Autodesk Fusion 360 part; units mm, degrees
note: some values were not read from the file. Set by a fixed rule: which sketch regions a step uses.
(part 2 of 2)
extrude "Extrude7" add sketch "Sketch3" against normal blind 4 contours A0 | A2 | A4 | A6 bodies 11 in component "bottom"
sketch "Sketch4" plane through (0, 0, 17.5) normal (0, 0, -1) x (1, 0, 0) in component "bottom"
  line L0 (73, -115.5) -> (73, -139.5)
  line L1 (73, -139.5) -> (27, -139.5)
  line L2 (27, -139.5) -> (27, -115.5)
  line L3 (27, -115.5) -> (73, -115.5)
  line L4 (25, -141.5) -> (75, -141.5)
  line L5 (75, -141.5) -> (75, -113.5)
  line L6 (75, -113.5) -> (25, -113.5)
  line L7 (25, -113.5) -> (25, -141.5)
  circle A0 centre (30.95, -119.25) radius 2.5
  circle A1 centre (30.95, -119.25) radius 1.4
  circle A2 centre (69.05, -119.25) radius 2.5
  circle A3 centre (69.05, -119.25) radius 1.4
  circle A4 centre (69.05, -135.75) radius 2.5
  circle A5 centre (69.05, -135.75) radius 1.4
  circle A6 centre (30.95, -135.75) radius 2.5
  circle A7 centre (30.95, -135.75) radius 1.4
extrude "Extrude8" add sketch "Sketch4" against normal blind 7 contours L0 L1 L2 L3 bodies 12 in component "bottom"
extrude "Extrude9" add sketch "Sketch4" against normal blind 4 contours A0 | A2 | A4 | A6 bodies 12 in component "bottom"
extrude "Extrude10" add sketch "Sketch1 (2)" against normal blind 4 contours A99 A102 L91 A128 A132 L174 | A99 L88 A100 A128 A134 L175 | A127 A128 L174 A137 L175 | A128 A132 A133 A134 L173 L174 L175 L176 | A127 A128 L174 A137 L175 | A101 L90 A102 A132 A133 L173 | A131 A132 L173 A136 L174 | A131 A132 L173 A136 L174 | A129 A134 L175 A138 L176 | A129 A134 L175 A138 L176 | A100 L89 A101 A133 A134 L176 | A127 A137 | A127 A137 | A130 A133 A135 L173 L176 | A130 A133 A135 L173 L176 | A131 A136 | A131 A136 | A129 A138 | A129 A138 | A130 A135 | A130 A135 | L93 L96 L136 L137 | L93 L96 L99 L100 L104 L115 | L93 L115 L136 L137 | L96 L104 L136 L137 | L93 L113 L115 L116 L117 | L93 L100 L113 L114 L115 L117 | L103 L109 L112 L116 L119 L123 L128 L132 L134 L135 L136 L137 L138 L139 L140 L141 | L96 L99 L102 L104 L105 | L96 L102 L103 L104 L106 | L93 L111 L112 L113 L117 | L93 L100 L110 L111 L113 L117 | L96 L99 L102 L107 L172 | L96 L102 L106 L107 L108 L109 | L93 L111 L138 L139 | L93 L94 L100 L101 L111 L120 | L95 L96 L98 L99 L127 L172 | L96 L108 L134 L135 | L93 L94 L138 L139 | L95 L96 L134 L135 | L94 L120 L138 L139 | L95 L127 L134 L135 | L94 L118 L119 L120 L122 | L94 L101 L118 L120 L121 L122 | L95 L127 L128 L129 L133 | L95 L98 L126 L127 L129 L133 | L94 L118 L122 L123 L124 | L94 L101 L118 L122 L124 L125 | L95 L129 L131 L132 L133 | L95 L98 L129 L130 L131 L133 | L94 L95 L124 L140 | L94 L95 L98 L101 L124 L131 | L95 L131 L140 L141 | L154 L155 L156 L157 | L159 L160 L162 L163 bodies 2 3 4 5 6 7 8 9 10 11 12 in component "bottom"
sketch "Sketch5" plane through (175, 0, 0) normal (1, 0, 0) x (0, 1, 0) in component "bottom"
  line L0 (6, 56.5) -> (6, -2.5)
  line L1 (6, -2.5) -> (139, -2.5)
  line L2 (139, -2.5) -> (139, 56.5)
  line L3 (126, -17.5) -> (96, -17.5) construction
  line L4 (96, -17.5) -> (111, -17.5) construction
  line L5 (111, -17.5) -> (111, 50.5) construction
  line L6 (139, 56.5) -> (6, 56.5)
  line L7 (141.5, 52.5) -> (113.5, 52.5)
  line L8 (113.5, 52.5) -> (141.5, 52.5)
  line L9 (0, 52.5) -> (6.7574, 52.5)
  line L10 (6.4384, 52.5) -> (138.5616, 52.5)
  line L11 (138.2426, 52.5) -> (145, 52.5)
  line L12 (138.2426, 52.5) -> (145, 52.5)
  line L13 (138.5616, 52.5) -> (6.4384, 52.5)
  line L14 (0, 52.5) -> (6.7574, 52.5)
  line L15 (30.523, 52.5) -> (6.123, 52.5)
  line L16 (6.123, 52.5) -> (13.123, 52.5)
  line L17 (13.123, 52.5) -> (30.523, 52.5)
  line L18 (30.523, 52.5) -> (13.123, 52.5)
  line L19 (13.123, 52.5) -> (6.123, 52.5)
  line L20 (6.123, 52.5) -> (30.523, 52.5)
  line L21 (70.523, 52.5) -> (63.523, 52.5)
  line L22 (63.523, 52.5) -> (46.123, 52.5)
  line L23 (46.123, 52.5) -> (70.523, 52.5)
  line L24 (46.123, 52.5) -> (63.523, 52.5)
  line L25 (63.523, 52.5) -> (70.523, 52.5)
  line L26 (70.523, 52.5) -> (46.123, 52.5)
  line L27 (80.5, 52.5) -> (108.5, 52.5)
  line L28 (108.5, 52.5) -> (80.5, 52.5)
  line L29 (111, 50.5) -> (111, 52.5)
  line L30 (111, 52.5) -> (111, 25.5)
  circle A0 centre (126, 25.5) radius 3.2
  line L31 (105, 22) -> (97, 22)
  line L32 (95, 24) -> (95, 27)
  line L33 (97, 29) -> (105, 29)
  line L34 (107, 27) -> (107, 24)
  line L35 (107, 22) -> (95, 29) construction
  line L36 (101, 25.5) -> (91, 25.5) construction
  line L37 (101, 25.5) -> (111, 25.5) construction
  circle A1 centre (91, 25.5) radius 1.65
  circle A2 centre (111, 25.5) radius 1.65
  arc A3 (105, 22) -> (107, 24) centre (105, 24) ccw
  arc A4 (107, 27) -> (105, 29) centre (105, 27) ccw
  arc A5 (95, 24) -> (97, 22) centre (97, 24) ccw
  arc A6 (97, 29) -> (95, 27) centre (97, 27) ccw
  line L38 (111, 25.5) -> (126, 25.5) construction
  point P0 (126, -17.5)
  point P1 (96, -17.5)
  point P2 (95, 22)
  point P3 (107, 29)
  dimension "d207" = 27
  dimension "d220" = 6.4
  dimension "d221" = 12
  dimension "d222" = 7
  dimension "d223" = 10
  dimension "d224" = 10
  dimension "d225" = 3.3
  dimension "d226" = 3.3
  dimension "d227" = 2
  dimension "d228" = 15
  constraint coincident P0 L3.start
  constraint coincident P1 L3.end
  constraint midpoint L3 L4.end
  constraint coincident L10 L29.end
  constraint perpendicular L10 L29
  constraint collinear L5 L29
  constraint horizontal L31
  constraint vertical L32
  constraint horizontal L33
  constraint vertical L34
  constraint midpoint L35 L36.start
  constraint perpendicular L32 L36
  constraint perpendicular L34 L37
  constraint coincident L36.end A1.centre
  constraint coincident L30.end L37.end
  constraint coincident L35.start L31
  constraint coincident L35.start L34
  constraint tangent L31 A3
  constraint tangent L34 A3
  constraint coincident P3 L33
  constraint coincident P3 L34
  constraint tangent L33 A4
  constraint tangent L34 A4
  constraint equal A3 A4
  constraint coincident P2 L31
  constraint coincident P2 L32
  constraint tangent L31 A5
  constraint tangent L32 A5
  constraint equal A3 A5
  constraint coincident L35.end L33
  constraint coincident L35.end L32
  constraint tangent L33 A6
  constraint tangent L32 A6
  constraint equal A3 A6
  constraint parallel L37 L38
  constraint coincident A0.centre L38.end
  constraint perpendicular L27 L30
  measures "d207" distance of L29.end L30.end
  measures "d220" diameter of A0
  measures "d221" distance of L35.start P2
  measures "d222" distance of L35.start P3
  measures "d223" distance of L36.start L36.end
  measures "d224" distance of L36.start L30.end
  measures "d225" diameter of A1
  measures "d226" diameter of A2
  measures "d227" radius of A3
  measures "d228" distance of L30.end A0.centre
extrude "Extrude12" add sketch "Sketch4" sketch "Sketch3" along normal blind 4 contours L0 L1 L2 L3 | L4 L5 L6 L7 | A0 | A2 | A4 | A6 of sketch 2 contours L0 L1 L2 L3 | L4 L5 L6 L7 | A0 | A2 | A4 | A6 bodies 2 in component "bottom"
extrude "Extrude13" cut 4 faces at (67.0569, 86.9948, 21.5) (67.0569, 103.4948, 21.5) (29.1251, 85.1561, 21.5) (29.1251, 101.6561, 21.5) along direction (0, 0, -1) blind 4 on bodies 2 bodies 2 in component "bottom"
extrude "Extrude14" cut 1 faces at (44.4008, 96.8884, 24.5) along direction (0, 0, -1) blind 4 on bodies 2 bodies 2 in component "bottom"
extrude "Extrude15" cut 1 faces at (44.4008, 125.1116, 24.5) along direction (0, 0, -1) blind 4 on bodies 2 bodies 2 in component "bottom"
extrude "Extrude16" cut 4 faces at (33.0688, 119.4438, 21.5) (33.0163, 135.2426, 21.5) (67.0569, 119.9948, 21.5) (66.9837, 136.2574, 21.5) along direction (0, 0, -1) blind 4 on bodies 2 bodies 2 in component "bottom"
extrude "Extrude17" cut 1 faces at (141, 75.8333, 56.5) along direction (0, 0, -1) blind 1.5 on bodies 2 bodies 2 in component "bottom"
extrude "Extrude18" cut 1 faces at (58.8128, 145, 34.1667) along direction (0, 1, 0) blind 2.5 on bodies 2 bodies 2 in component "bottom"
extrude "Extrude19" cut 1 faces at (170, 94.5205, 15.8333) along direction (1, 0, 0) blind 2.5 on bodies 2 bodies 2 in component "bottom"
extrude "Extrude20" cut 1 faces at (0, 50.4795, 34.1667) along direction (-1, 0, 0) blind 2.5 on bodies 2 bodies 2 in component "bottom"
extrude "Extrude21" cut 1 faces at (111.1872, 0, 34.1667) along direction (0, -1, 0) blind 2.5 on bodies 2 bodies 2 in component "bottom"
extrude "Extrude22" cut 2 faces at (36.4, 13.123, 35.8333) (63.6, 13.123, 35.8333) along direction (0, -1, 0) blind 2 on bodies 2 bodies 2 in component "bottom"
extrude "Extrude23" cut 2 faces at (63.6, 63.523, 35.8333) (36.4, 63.523, 35.8333) along direction (0, 1, 0) blind 2 on bodies 2 bodies 2 in component "bottom"
extrude "Extrude24" cut 2 faces at (24.8, 52.5896, 35.8333) (24.8, 17.5896, 19.1667) along direction (-1, 0, 0) blind 2 on bodies 2 bodies 2 in component "bottom"
extrude "Extrude25" cut 2 faces at (75.2, 17.5896, 19.1667) (75.2, 52.5896, 35.8333) along direction (1, 0, 0) blind 2 on bodies 2 bodies 2 in component "bottom"
fillet "Fillet3" radius 8 8 edges at (67.5, 65.523, 52.5) (32.5, 65.523, 52.5) (22.8, 55.823, 52.5) (22.8, 20.823, 52.5) (32.5, 11.123, 52.5) (77.2, 20.823, 52.5) (67.5, 11.123, 52.5) (77.2, 55.823, 52.5) on bodies 2 in component "bottom"
fillet "Fillet4" radius 2 8 edges at (50, 113.5, 13.5) (75, 127.5, 13.5) (50, 141.5, 13.5) (25, 127.5, 13.5) (25, 94.5, 13.5) (50, 80.5, 13.5) (50, 108.5, 13.5) (75, 94.5, 13.5) on bodies 2 in component "bottom"
fillet "Fillet5" radius 6 8 edges at (85, 150, 55) (171.7782, 146.7782, 55) (175, 72.5, 55) (171.7782, -1.7782, 55) (85, -5, 55) (-1.7782, -1.7782, 55) (-5, 72.5, 55) (-1.7782, 146.7782, 55) on bodies 2 in component "bottom"
fillet "Fillet6" radius 2 8 edges at (50, 82.5, 55) (27, 94.5, 55) (50, 106.5, 55) (73, 94.5, 55) (50, 115.5, 55) (27, 127.5, 55) (50, 139.5, 55) (73, 127.5, 55) on bodies 2 in component "bottom"
extrude "Extrude6'" add 9 faces at (98.1986, 29.7171, -15.5) (125.1986, 29.7171, -15.5) (98.2222, 58.415, -15.5) (125.2222, 58.415, -15.5) (151.6624, 57.1856, -15.5) (153.6175, 30.3228, -15.5) (125.1986, 2.7171, -15.5) (153.6175, 3.6077, -15.5) (98.1986, 2.7171, -15.5) along direction (0, 0, -1) blind 2 on bodies 1 bodies 1 in component "Lid"
sketch "Sketch2 (2)" plane through (0, 0, -15) normal (0, 0, 1) x (-1, 0, 0) in component "Lid"
  arc A0 (-63, -19.323) -> (-61, -21.323) centre (-61, -19.323) ccw
  line L0 (-63, -19.323) -> (-63, -12.323)
  arc A1 (-61, -10.323) -> (-63, -12.323) centre (-61, -12.323) ccw
  line L1 (-61, -10.323) -> (-54, -10.323)
  arc A2 (-52, -12.323) -> (-54, -10.323) centre (-54, -12.323) ccw
  line L2 (-52, -12.323) -> (-52, -19.323)
  arc A3 (-54, -21.323) -> (-52, -19.323) centre (-54, -19.323) ccw
  line L3 (-54, -21.323) -> (-61, -21.323)
  arc A4 (-78, -19.323) -> (-76, -21.323) centre (-76, -19.323) ccw
  line L4 (-78, -19.323) -> (-78, -12.323)
  arc A5 (-76, -10.323) -> (-78, -12.323) centre (-76, -12.323) ccw
  line L5 (-76, -10.323) -> (-69, -10.323)
  arc A6 (-67, -12.323) -> (-69, -10.323) centre (-69, -12.323) ccw
  line L6 (-67, -12.323) -> (-67, -19.323)
  arc A7 (-69, -21.323) -> (-67, -19.323) centre (-69, -19.323) ccw
  line L7 (-69, -21.323) -> (-76, -21.323)
  arc A8 (-48, -19.323) -> (-46, -21.323) centre (-46, -19.323) ccw
  line L8 (-48, -19.323) -> (-48, -12.323)
  arc A9 (-46, -10.323) -> (-48, -12.323) centre (-46, -12.323) ccw
  line L9 (-46, -10.323) -> (-39, -10.323)
  arc A10 (-37, -12.323) -> (-39, -10.323) centre (-39, -12.323) ccw
  line L10 (-37, -12.323) -> (-37, -19.323)
  arc A11 (-39, -21.323) -> (-37, -19.323) centre (-39, -19.323) ccw
  line L11 (-39, -21.323) -> (-46, -21.323)
  circle A12 centre (-1.7574, -143.2426) radius 1.65
  arc A13 (-78, -64.323) -> (-76, -66.323) centre (-76, -64.323) ccw
  line L12 (-78, -64.323) -> (-78, -57.323)
  arc A14 (-76, -55.323) -> (-78, -57.323) centre (-76, -57.323) ccw
  line L13 (-76, -55.323) -> (-69, -55.323)
  arc A15 (-67, -57.323) -> (-69, -55.323) centre (-69, -57.323) ccw
  line L14 (-67, -57.323) -> (-67, -64.323)
  arc A16 (-69, -66.323) -> (-67, -64.323) centre (-69, -64.323) ccw
  line L15 (-69, -66.323) -> (-76, -66.323)
  arc A17 (-33, -49.323) -> (-31, -51.323) centre (-31, -49.323) ccw
  line L16 (-33, -49.323) -> (-33, -42.323)
  arc A18 (-31, -40.323) -> (-33, -42.323) centre (-31, -42.323) ccw
  line L17 (-31, -40.323) -> (-24, -40.323)
  arc A19 (-22, -42.323) -> (-24, -40.323) centre (-24, -42.323) ccw
  line L18 (-22, -42.323) -> (-22, -49.323)
  arc A20 (-24, -51.323) -> (-22, -49.323) centre (-24, -49.323) ccw
  line L19 (-24, -51.323) -> (-31, -51.323)
  circle A21 centre (-113.5, -77.8144) radius 1.45
  circle A22 centre (-168.2426, -1.7574) radius 1.65
  arc A23 (-48, -49.323) -> (-46, -51.323) centre (-46, -49.323) ccw
  line L20 (-48, -49.323) -> (-48, -42.323)
  arc A24 (-46, -40.323) -> (-48, -42.323) centre (-46, -42.323) ccw
  line L21 (-46, -40.323) -> (-39, -40.323)
  arc A25 (-37, -42.323) -> (-39, -40.323) centre (-39, -42.323) ccw
  line L22 (-37, -42.323) -> (-37, -49.323)
  arc A26 (-39, -51.323) -> (-37, -49.323) centre (-39, -49.323) ccw
  line L23 (-39, -51.323) -> (-46, -51.323)
  circle A27 centre (-125.5, -65.3144) radius 3.75
  line L24 (-138.5, -101.6644) -> (-138.5, -86.6644)
  line L25 (-138.5, -86.6644) -> (-112.5, -86.6644)
  line L26 (-112.5, -86.6644) -> (-112.5, -101.6644)
  line L27 (-112.5, -101.6644) -> (-138.5, -101.6644)
  circle A28 centre (-1.7574, -1.7574) radius 1.65
  arc A29 (-48, -64.323) -> (-46, -66.323) centre (-46, -64.323) ccw
  line L28 (-48, -64.323) -> (-48, -57.323)
  arc A30 (-46, -55.323) -> (-48, -57.323) centre (-46, -57.323) ccw
  line L29 (-46, -55.323) -> (-39, -55.323)
  arc A31 (-37, -57.323) -> (-39, -55.323) centre (-39, -57.323) ccw
  line L30 (-37, -57.323) -> (-37, -64.323)
  arc A32 (-39, -66.323) -> (-37, -64.323) centre (-39, -64.323) ccw
  line L31 (-39, -66.323) -> (-46, -66.323)
  arc A33 (-63, -64.323) -> (-61, -66.323) centre (-61, -64.323) ccw
  line L32 (-63, -64.323) -> (-63, -57.323)
  arc A34 (-61, -55.323) -> (-63, -57.323) centre (-61, -57.323) ccw
  line L33 (-61, -55.323) -> (-54, -55.323)
  arc A35 (-52, -57.323) -> (-54, -55.323) centre (-54, -57.323) ccw
  line L34 (-52, -57.323) -> (-52, -64.323)
  arc A36 (-54, -66.323) -> (-52, -64.323) centre (-54, -64.323) ccw
  line L35 (-54, -66.323) -> (-61, -66.323)
  circle A37 centre (-137.5, -77.8144) radius 1.45
  arc A38 (-63, -34.323) -> (-61, -36.323) centre (-61, -34.323) ccw
  line L36 (-63, -34.323) -> (-63, -27.323)
  arc A39 (-61, -25.323) -> (-63, -27.323) centre (-61, -27.323) ccw
  line L37 (-61, -25.323) -> (-54, -25.323)
  arc A40 (-52, -27.323) -> (-54, -25.323) centre (-54, -27.323) ccw
  line L38 (-52, -27.323) -> (-52, -34.323)
  arc A41 (-54, -36.323) -> (-52, -34.323) centre (-54, -34.323) ccw
  line L39 (-54, -36.323) -> (-61, -36.323)
  arc A42 (-78, -34.323) -> (-76, -36.323) centre (-76, -34.323) ccw
  line L40 (-78, -34.323) -> (-78, -27.323)
  arc A43 (-76, -25.323) -> (-78, -27.323) centre (-76, -27.323) ccw
  line L41 (-76, -25.323) -> (-69, -25.323)
  arc A44 (-67, -27.323) -> (-69, -25.323) centre (-69, -27.323) ccw
  line L42 (-67, -27.323) -> (-67, -34.323)
  arc A45 (-69, -36.323) -> (-67, -34.323) centre (-69, -34.323) ccw
  line L43 (-69, -36.323) -> (-76, -36.323)
  arc A46 (-33, -19.323) -> (-31, -21.323) centre (-31, -19.323) ccw
  line L44 (-33, -19.323) -> (-33, -12.323)
  arc A47 (-31, -10.323) -> (-33, -12.323) centre (-31, -12.323) ccw
  line L45 (-31, -10.323) -> (-24, -10.323)
  arc A48 (-22, -12.323) -> (-24, -10.323) centre (-24, -12.323) ccw
  line L46 (-22, -12.323) -> (-22, -19.323)
  arc A49 (-24, -21.323) -> (-22, -19.323) centre (-24, -19.323) ccw
  line L47 (-24, -21.323) -> (-31, -21.323)
  circle A50 centre (-137.5, -104.6144) radius 1.45
  arc A51 (-63, -49.323) -> (-61, -51.323) centre (-61, -49.323) ccw
  line L48 (-63, -49.323) -> (-63, -42.323)
  arc A52 (-61, -40.323) -> (-63, -42.323) centre (-61, -42.323) ccw
  line L49 (-61, -40.323) -> (-54, -40.323)
  arc A53 (-52, -42.323) -> (-54, -40.323) centre (-54, -42.323) ccw
  line L50 (-52, -42.323) -> (-52, -49.323)
  arc A54 (-54, -51.323) -> (-52, -49.323) centre (-54, -49.323) ccw
  line L51 (-54, -51.323) -> (-61, -51.323)
  arc A55 (-78, -49.323) -> (-76, -51.323) centre (-76, -49.323) ccw
  line L52 (-78, -49.323) -> (-78, -42.323)
  arc A56 (-76, -40.323) -> (-78, -42.323) centre (-76, -42.323) ccw
  line L53 (-76, -40.323) -> (-69, -40.323)
  arc A57 (-67, -42.323) -> (-69, -40.323) centre (-69, -42.323) ccw
  line L54 (-67, -42.323) -> (-67, -49.323)
  arc A58 (-69, -51.323) -> (-67, -49.323) centre (-69, -49.323) ccw
  line L55 (-69, -51.323) -> (-76, -51.323)
  circle A59 centre (-168.2426, -143.2426) radius 1.65
  arc A60 (-33, -34.323) -> (-31, -36.323) centre (-31, -34.323) ccw
  line L56 (-33, -34.323) -> (-33, -27.323)
  arc A61 (-31, -25.323) -> (-33, -27.323) centre (-31, -27.323) ccw
  line L57 (-31, -25.323) -> (-24, -25.323)
  arc A62 (-22, -27.323) -> (-24, -25.323) centre (-24, -27.323) ccw
  line L58 (-22, -27.323) -> (-22, -34.323)
  arc A63 (-24, -36.323) -> (-22, -34.323) centre (-24, -34.323) ccw
  line L59 (-24, -36.323) -> (-31, -36.323)
  circle A64 centre (-98.5, -11.3144) radius 3.75
  line L60 (-106, -136.7179) -> (-118.0203, -130.3379)
  arc A65 (-118.0203, -130.3379) -> (-118.0203, -124.6621) centre (-125.5, -127.5) ccw
  line L61 (-118.0203, -124.6621) -> (-106, -118.2821)
  line L62 (-106, -118.2821) -> (-106, -136.7179)
  circle A66 centre (-97, -139.5) radius 1.65
  line L63 (-108.133, -117.15) -> (-118.9579, -122.8955)
  arc A67 (-118.9579, -122.8955) -> (-132.0421, -122.8955) centre (-125.5, -127.5) ccw
  line L64 (-132.0421, -122.8955) -> (-142.867, -117.15)
  line L65 (-142.867, -117.15) -> (-108.133, -117.15)
  circle A68 centre (-97, -115.5) radius 1.65
  line L66 (-118.9579, -132.1045) -> (-108.133, -137.85)
  line L67 (-108.133, -137.85) -> (-142.867, -137.85)
  line L68 (-142.867, -137.85) -> (-132.0421, -132.1045)
  arc A69 (-132.0421, -132.1045) -> (-118.9579, -132.1045) centre (-125.5, -127.5) ccw
  circle A70 centre (-152.5, -38.3144) radius 3.75
  line L69 (-145, -136.7179) -> (-145, -118.2821)
  line L70 (-145, -118.2821) -> (-132.9797, -124.6621)
  arc A71 (-132.9797, -124.6621) -> (-132.9797, -130.3379) centre (-125.5, -127.5) ccw
  line L71 (-132.9797, -130.3379) -> (-145, -136.7179)
  circle A72 centre (-125.5, -127.5) radius 6
  circle A73 centre (-152.5, -65.3144) radius 3.75
  circle A74 centre (-98.5, -38.3144) radius 3.75
  circle A75 centre (-125.5, -38.3144) radius 3.75
  circle A76 centre (-125.5, -11.3144) radius 3.75
  circle A77 centre (-152.5, -11.3144) radius 3.75
  line L72 (-90, -126) -> (-10, -126)
  line L73 (-10, -126) -> (-10, -129)
  line L74 (-10, -129) -> (-90, -129)
  line L75 (-90, -129) -> (-90, -126)
  arc A78 (-24, -66.323) -> (-22, -64.323) centre (-24, -64.323) ccw
  line L76 (-24, -66.323) -> (-31, -66.323)
  arc A79 (-33, -64.323) -> (-31, -66.323) centre (-31, -64.323) ccw
  line L77 (-33, -64.323) -> (-33, -57.323)
  arc A80 (-31, -55.323) -> (-33, -57.323) centre (-31, -57.323) ccw
  line L78 (-31, -55.323) -> (-24, -55.323)
  arc A81 (-22, -57.323) -> (-24, -55.323) centre (-24, -57.323) ccw
  line L79 (-22, -57.323) -> (-22, -64.323)
  circle A82 centre (-98.5, -65.3144) radius 3.75
  line L80 (-90, -93) -> (-10, -93)
  line L81 (-10, -93) -> (-10, -96)
  line L82 (-10, -96) -> (-90, -96)
  line L83 (-90, -96) -> (-90, -93)
  arc A83 (-48, -34.323) -> (-46, -36.323) centre (-46, -34.323) ccw
  line L84 (-48, -34.323) -> (-48, -27.323)
  arc A84 (-46, -25.323) -> (-48, -27.323) centre (-46, -27.323) ccw
  line L85 (-46, -25.323) -> (-39, -25.323)
  arc A85 (-37, -27.323) -> (-39, -25.323) centre (-39, -27.323) ccw
  line L86 (-37, -27.323) -> (-37, -34.323)
  arc A86 (-39, -36.323) -> (-37, -34.323) centre (-39, -34.323) ccw
  line L87 (-39, -36.323) -> (-46, -36.323)
  circle A87 centre (-113.5, -104.6144) radius 1.45
  circle A88 centre (-160, -115.5) radius 1.65
  circle A89 centre (-160, -139.5) radius 1.65
  arc A90 (-6, -150) -> (5, -139) centre (-6, -139) ccw
  line L88 (5, -139) -> (5, -6)
  arc A91 (5, -6) -> (-6, 5) centre (-6, -6) ccw
  line L89 (-6, 5) -> (-164, 5)
  arc A92 (-164, 5) -> (-175, -6) centre (-164, -6) ccw
  line L90 (-175, -6) -> (-175, -139)
  arc A93 (-175, -139) -> (-164, -150) centre (-164, -139) ccw
  line L91 (-164, -150) -> (-6, -150)
  circle A94 centre (-98.5, -57.5144) radius 1.45
  circle A95 centre (-125.5, -57.5144) radius 1.45
  circle A96 centre (-152.5, -57.5144) radius 1.45
  circle A97 centre (-125.5, -30.5144) radius 1.45
  circle A98 centre (-98.5, -30.5144) radius 1.45
  circle A99 centre (-152.5, -30.5144) radius 1.45
  circle A100 centre (-152.5, -3.5144) radius 1.45
  circle A101 centre (-125.5, -3.5144) radius 1.45
  circle A102 centre (-98.5, -3.5144) radius 1.45
extrude "Extrude7'" cut sketch "Sketch2 (2)" against normal blind 2 contours A94 | A95 | A96 | A97 | A98 | A99 | A100 | A101 | A102 bodies 1 in component "Lid"
extrude "Extrude26" add 1 faces at (58.8128, 147.5, 34.1667) along direction (0, -1, 0) blind 4 on bodies 2 bodies 2 in component "bottom"
extrude "Extrude27" add 1 faces at (-2.5, 50.4795, 34.1667) along direction (1, 0, 0) blind 3 on bodies 2 bodies 2 in component "bottom"
extrude "Extrude28" add 1 faces at (111.1872, -2.5, 34.1667) along direction (0, 1, 0) blind 3 on bodies 2 bodies 2 in component "bottom"
extrude "Extrude29" add 1 faces at (172.5, 94.5205, 15.8333) along direction (-1, 0, 0) blind 3 on bodies 2 bodies 2 in component "bottom"
sketch "Sketch6" plane through (175, 72.5, 25) normal (1, 0, 0) x (0, 1, 0) in component "bottom"
extrude "Extrude30" cut sketch "Sketch5" against normal blind 9 contours A0 | L31 L32 L33 L34 A3 A4 A5 A6 | A1 | A2 bodies 2 in component "bottom"
sketch "Sketch7" plane through (73, 0, 0) normal (-1, 0, 0) x (0, -1, 0) in component "bottom"
  line L0 (-82.5, 53) -> (-106.5, 53)
  line L1 (-106.5, 53) -> (-106.5, 20.5)
  line L2 (-106.5, 20.5) -> (-82.5, 20.5)
  line L3 (-82.5, 20.5) -> (-82.5, 53)
  line L4 (-94.5, 53) -> (-94.5, 43) construction
  line L5 (-139.5, 53) -> (-115.5, 53)
  line L6 (-127.5, 53) -> (-127.5, 43) construction
  circle A0 centre (-127.5, 43) radius 2.45
  line L7 (-127.5, 43) -> (-129.6, 43) construction
  line L8 (-129.6, 43) -> (-129.6, 44.2619)
  line L9 (-129.6, 43) -> (-129.6, 41.7381)
  circle A1 centre (-94.5, 43) radius 3
  line L10 (-94.5, 43) -> (-100.9, 43) construction
  circle A2 centre (-100.9, 43) radius 1.2
  dimension "d231" = 10
  dimension "d233" = 10
  dimension "d234" = 4.9
  dimension "d235" = 2.1
  dimension "d236" = 6
  dimension "d237" = 6.4
  dimension "d238" = 2.4
  constraint midpoint L0 L4.start
  constraint perpendicular L0 L4
  constraint midpoint L5 L6.start
  constraint perpendicular L5 L6
  constraint coincident L6.end A0.centre
  constraint perpendicular L6 L7
  constraint coincident A0 L8.end
  constraint perpendicular L7 L8
  constraint coincident A0 L9.end
  constraint perpendicular L7 L9
  constraint coincident L4.end A1.centre
  constraint perpendicular L4 L10
  constraint coincident L10.end A2.centre
  measures "d231" distance of L4.start L4.end
  measures "d233" distance of L6.start L6.end
  measures "d234" diameter of A0
  measures "d235" distance of L6.end L7.end
  measures "d236" diameter of A1
  measures "d237" distance of L4.end L10.end
  measures "d238" diameter of A2
extrude "Extrude31" cut sketch "Sketch7" against normal blind 4 contours A0 L8 L9 | A1 picked at (-126.5752, 42.8824) bodies 2 in component "bottom"
sketch "Sketch8" plane through (75, 0, 0) normal (1, 0, 0) x (0, 1, 0) in component "bottom"
  circle A0 centre (94.5, 43) radius 3
  line L0 (80.5, 15.5) -> (108.5, 15.5)
  line L1 (108.5, 15.5) -> (108.5, 52.5)
  line L2 (108.5, 52.5) -> (80.5, 52.5)
  line L3 (80.5, 52.5) -> (80.5, 15.5)
  circle A1 centre (100.9, 43) radius 1.2
extrude "Extrude32" cut sketch "Sketch8" against normal blind 1.5 contours A1 bodies 2 in component "bottom"
sketch "Sketch1 (3)" plane through (169.5, 0, 0) normal (-1, 0, 0) x (0, -1, 0)
  circle A0 centre (-91, 25.5) radius 1.65
  circle A1 centre (-111, 25.5) radius 1.65
  line L0 (-105, 29) -> (-97, 29)
  arc A2 (-95, 27) -> (-97, 29) centre (-97, 27) ccw
  line L1 (-95, 27) -> (-95, 24)
  arc A3 (-97, 22) -> (-95, 24) centre (-97, 24) ccw
  line L2 (-97, 22) -> (-105, 22)
  arc A4 (-107, 24) -> (-105, 22) centre (-105, 24) ccw
  line L3 (-107, 24) -> (-107, 27)
  arc A5 (-105, 29) -> (-107, 27) centre (-105, 27) ccw
  circle A6 centre (-126, 25.5) radius 3.2
  line L4 (-6.5967, -2.5) -> (-6.5967, 52.5)
  line L5 (-6.5967, 52.5) -> (-138.4033, 52.5)
  line L6 (-138.4033, 52.5) -> (-138.4033, -2.5)
  line L7 (-138.4033, -2.5) -> (-6.5967, -2.5)
  circle A7 centre (-126, 25.5) radius 6
  dimension "d243" = 12
  constraint concentric A6 A7
  measures "d243" diameter of A7
extrude "Extrude33" cut sketch "Sketch1 (3)" against normal blind 4 contours A7 bodies 2 in component "bottom"
sketch "Sketch2 (3)" plane through (169.5, 0, 0) normal (-1, 0, 0) x (0, -1, 0)
  circle A0 centre (-126, 25.5) radius 6
  circle A1 centre (-91, 25.5) radius 1.65
  circle A2 centre (-111, 25.5) radius 1.65
  line L0 (-105, 29) -> (-97, 29)
  arc A3 (-95, 27) -> (-97, 29) centre (-97, 27) ccw
  line L1 (-95, 27) -> (-95, 24)
  arc A4 (-97, 22) -> (-95, 24) centre (-97, 24) ccw
  line L2 (-97, 22) -> (-105, 22)
  arc A5 (-107, 24) -> (-105, 22) centre (-105, 24) ccw
  line L3 (-107, 24) -> (-107, 27)
  arc A6 (-105, 29) -> (-107, 27) centre (-105, 27) ccw
  line L4 (-6.5967, -2.5) -> (-6.5967, 52.5)
  line L5 (-6.5967, 52.5) -> (-138.4033, 52.5)
  line L6 (-138.4033, 52.5) -> (-138.4033, -2.5)
  line L7 (-138.4033, -2.5) -> (-6.5967, -2.5)
  line L8 (-86, 21) -> (-116, 21)
  line L9 (-116, 21) -> (-116, 30)
  line L10 (-116, 30) -> (-86, 30)
  line L11 (-86, 30) -> (-86, 21)
  line L12 (-86, 21) -> (-116, 30) construction
  line L13 (-95.5858, 22.5858) -> (-106.4142, 28.4142) construction
  dimension "d246" = 30
  dimension "d247" = 9
  constraint horizontal L8
  constraint vertical L9
  constraint horizontal L10
  constraint vertical L11
  constraint midpoint A4 L13.start
  constraint midpoint A6 L13.end
  constraint midpoint L12 L13
  measures "d246" distance of L8.start L8.end
  measures "d247" distance of L8.start L10.end
extrude "Extrude34" cut sketch "Sketch2 (3)" against normal blind 4 contours L8 L9 L10 L11 bodies 2 in component "bottom"
component "Lid" placed x (1, 0, 0) y (0, 1, 0) z (0, 0, 1) at (0, 0, 0)
component "bottom" placed x (1, 0, 0) y (0, 1, 0) z (0, 0, 1) at (0, 0, 0)
